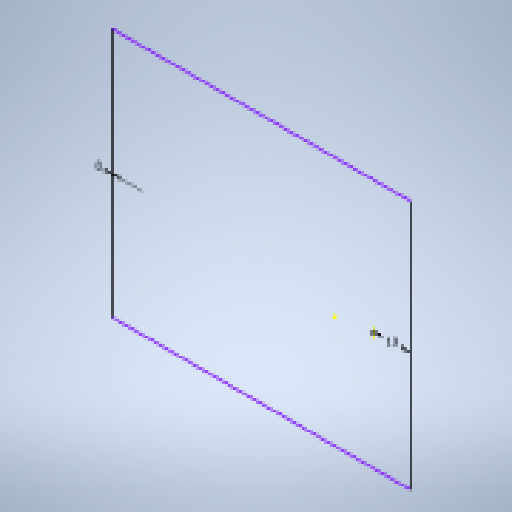
# Autodesk Inventor part: collectballLR
Saved by Autodesk Inventor 2023.2 (Build 272271030, 271C)
## iProperties
Created: 2023-06-21
Part Number: collectballLR
Material: Generic
Document SubType Name: Modeling
Designer: kao91
Density: 1 g/cm^3
Appearance: Default
Author: kao91
Autodesk Inventor part; units mm, degrees
ref_plane "YZ Plane" through (0, 0, 0) normal (1, 0, 0) x (0, 1, 0)
ref_plane "XZ Plane" through (0, 0, 0) normal (0, 1, 0) x (-1, 0, 0)
ref_plane "XY Plane" through (0, 0, 0) normal (0, 0, 1) x (1, 0, 0)
sketch "Sketch1" plane through (0, 0, 0) normal (0, 0, 1) x (1, 0, 0)
  line L0 (-54.0478, -39.25) -> (19.9951, -39.25)
  line L1 (-60.0049, 0) -> (-60.0049, 3) projected
  line L2 (9.9951, 0) -> (9.9951, 3) projected
  line L3 (9.9951, 0) -> (-0.0048, 0) projected
  line L4 (-0.0048, 0) -> (-0.0048, 3) projected
  line L5 (9.9951, 3) -> (-0.0048, 3) projected
  line L6 (9.9952, 0) -> (9.9952, 3) projected
  line L7 (9.9951, 0) -> (19.9951, 0)
  line L8 (19.9951, 3) -> (10.1225, 3)
  line L9 (19.9951, -39.25) -> (19.9951, 0)
  line L10 (19.9951, 3) -> (19.9951, 63)
  arc A0 (-54.0478, -39.25) -> (-15.3503, 63) centre (-67.8068, 24.405) ccw
  line L11 (19.9951, 63) -> (-15.3503, 63)
  circle A1 centre (-67.8068, 24.405) radius 25
  circle A2 centre (-67.8068, 7.905) radius 9
  circle A3 centre (-52.8068, 24.405) radius 11
  circle A4 centre (-5.5, -11.25) radius 2.0625 projected
  line L12 (-5.5, -11.25) -> (-5.5, -41.25)
  line L13 (10.1225, 3) -> (-0.0048, 3)
  line L14 (-0.0048, 0) -> (19.9951, 0)
  point P0 (9.9951, 1.5)
  point P1 (4.9951, 3)
  point P2 (10.1225, 3)
  point P3 (9.9951, 3)
  dimension "d5" = 50
  dimension "d6" = 40.125
  dimension "d7" = 35.3453
  dimension "d9" = 10
  dimension "d10" = 10
  dimension "d11" = 18
  dimension "d12" = 16.5
  dimension "d13" = 0
  dimension "d14" = 22
  dimension "d15" = 15
  dimension "d16" = 0
  dimension "d20" = 30
  dimension "d22" = 2
  dimension "d23" = 60
  constraints: 18 end point, 4 centre point, 3 horizontal, 3 perpendicular, 2 collinear, 2 midpoint, 2 point on circle, 1 coincident, 1 parallel, 1 other
  measures "d5" diameter of A1
  measures "d6" radial gap between concentric circles of A0 A1
  measures "d7" distance of L10.end L11.end
  measures "d9" distance between parallel lines of L2 L9
  measures "d10" distance between parallel lines of L2 L10
  measures "d11" diameter of A2
  measures "d12" distance of A1.centre A2.centre
  measures "d13" horizontal distance of A0.centre A2.centre
  measures "d14" diameter of A3
  measures "d15" distance of A3.centre A0.centre
  measures "d16" vertical distance of A0.centre A3.centre
  measures "d20" distance of L12.start L12.end
  measures "d22" distance from line of L12.end L0
  measures "d23" distance between parallel lines of L8 L11
extrude "Extrusion1" add sketch "Sketch1" along normal blind 3 contours A4 | A0 L11 L10 L8 L13 L5 L4 L3 L7 L9 L0 | L3 L4 L5 L2
body "Solid1"
